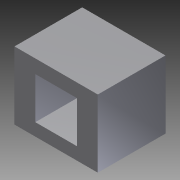
# Autodesk Inventor part: Wheel_axle_inner_spacer
Saved by Autodesk Inventor 2011 (Build 150239000, 239)
## iProperties
Created: 2013-01-31
Part Number: Wheel_axle_inner_spacer
Document SubType Name: Modeling
Designer: Christopher
Density: 1 g/cm^3
Author: Christopher
Autodesk Inventor part; units mm, degrees
ref_plane "YZ Plane" through (0, 0, 0) normal (1, 0, 0) x (0, 1, 0)
ref_plane "XZ Plane" through (0, 0, 0) normal (0, 1, 0) x (-1, 0, 0)
ref_plane "XY Plane" through (0, 0, 0) normal (0, 0, 1) x (1, 0, 0)
sketch "Sketch1" plane through (0, 0, 0) normal (0, 0, 1) x (1, 0, 0)
  line L0 (0, 0) -> (25.4, 0)
  line L1 (25.4, 0) -> (25.4, 20.6375)
  line L2 (25.4, 20.6375) -> (0, 20.6375)
  line L3 (0, 20.6375) -> (0, 0)
  line L4 (6.35, 3.81) -> (19.05, 3.81)
  line L5 (19.05, 3.81) -> (19.05, 16.51)
  line L6 (19.05, 16.51) -> (6.35, 16.51)
  line L7 (6.35, 16.51) -> (6.35, 3.81)
  point P0 (0, 10.3188)
  point P1 (12.7, 20.6375)
  dimension "d0" = 25.4
  dimension "d1" = 20.6375
  dimension "d22" = 12.7
  dimension "d23" = 12.7
  dimension "d24" = 6.35
  dimension "d25" = 4.1275
  constraints: 16 end point, 4 parallel, 2 horizontal, 2 midpoint, 2 perpendicular
  measures "d0" distance of L2.end L1.end
  measures "d1" distance of L1.end L0.end
  measures "d22" distance of L5.end L6.end
  measures "d23" distance of L4.end L5.end
  measures "d24" distance between parallel lines of L3 L7
  measures "d25" distance between parallel lines of L2 L6
extrude "Extrusion2" add sketch "Sketch1" against normal blind 20.6375
body "Solid2"
